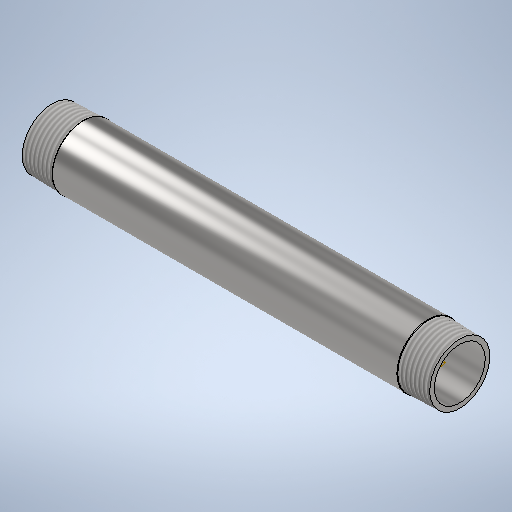
# Autodesk Inventor part: Threaded pipe_SGP._1ipt
Saved by Autodesk Inventor 2025.4 (Build 294407000, 407)
## iProperties
Created: 2026-06-08
Part Number: Threaded pipe_SGP._1ipt
Material: SS400
Document SubType Name: Modeling
Designer: huma2
Density: 7.98 g/cm^3
Appearance: 半つや出し
Manager: A_Shiramizu
Company: Eiko Engineering
length: 150.000 mm
Author: huma2
length: 200.000 mm
Comments: 免責事項 本3Dモデルは設計検討・参考用データです。寸法、形状、強度、材質、規格適合性、使用目的への適合性は保証しません。実際の設計・製作・使用にあたっては、利用者の責任でメーカー資料、規格、法令、現物確認、強度確認等を行ってください。 本データの使用・改変・流用・再配布により生じた損害、事故、不具合等について、作成者は一切責任を負いません。 Disclaimer This 3D model and related data are provided for reference and design study purposes only. The creator makes no warranty regarding dimensions, geometry, strength, material, standards compliance, or fitness for any particular purpose. Before actual design, fabrication, installation, purchase, or use, the user must verify all information, including actual products, manufacturer data, applicable standards, laws, and strength calculations. The creator shall not be liable for any damage, accident, defect, loss, or trouble arising from the use, modification, reuse, or redistribution of this data. Use of this data is entirely at the user's own risk.
Autodesk Inventor part; units mm, degrees
ref_plane "YZ Plane" through (0, 0, 0) normal (1, 0, 0) x (0, 1, 0)
ref_plane "XZ Plane" through (0, 0, 0) normal (0, 1, 0) x (-1, 0, 0)
ref_plane "XY Plane" through (0, 0, 0) normal (0, 0, 1) x (1, 0, 0)
sketch "スケッチ1" plane through (0, 0, 0) normal (0, 0, 1) x (1, 0, 0)
  line L0 (-110.39, 0) -> (110.39, 0)
  line L1 (-110.39, 0) -> (-110.39, 17)
  line L2 (-110.39, 17) -> (110.39, 17)
  line L3 (110.39, 0) -> (110.39, 17)
  line L4 (-110.39, 13.8) -> (110.39, 13.8)
  point P0 (0, 0)
  point P1 (0, 0)
  dimension "d0" = 34
  dimension "d1" = 3.2
  dimension "d2" = 220.78
  constraints: 10 end point, 2 point on line, 2 vertical, 1 coincident, 1 horizontal, 1 midpoint, 1 parallel
  measures "d0" diameter of L2 L0
  measures "d1" distance between parallel lines of L4 L2
  measures "d2" distance between parallel lines of L3 L1
revolve "回転1" add sketch "スケッチ1" angle 360 about axis through (-110.39, 0, 0) along (1, 0, 0) contours L1 L2 L3 L4
sketch "スケッチ2" plane through (0, 0, 0) normal (0, 0, 1) x (1, 0, 0)
  line L0 (-110.39, 17) -> (110.39, 17) projected
  line L1 (-110.39, -17) -> (-110.39, 17) projected
  line L2 (-110.39, 16.2998) -> (-93.6, 16.8245)
  line L3 (-93.6, 16.8245) -> (-93.296, 17)
  line L4 (-110.39, 0) -> (57.6085, 0)
  line L5 (-100, 16.6245) -> (-100, 0) construction
  point P0 (0, 0)
  dimension "d4" = 33.249
  dimension "d5" = 1.79
  dimension "d6" = 10.39
  dimension "d9" = 30
  dimension "d10" = 6.4
  constraints: 8 end point, 4 point on line, 1 horizontal, 1 midpoint, 1 perpendicular
  measures "d4" diameter of L5.start L4
  measures "d5" angle of L4 L2
  measures "d6" distance between parallel lines of L1 L5
  measures "d9" angle of L4 L3
  measures "d10" distance from line of L5 L2.end
revolve "回転2" cut sketch "スケッチ2" angle 360 about axis through (-110.39, 0, 0) along (1, 0, 0)
thread "ねじ1【手修正】" size "R 1" standard "JIS Taper" length 22.6
mirror "ミラー1" about plane through (0, 0, 0) normal (1, 0, 0) of "回転2"
thread "ねじ2【手修正】" size "R 1" standard "ISO Taper" length 23.2
ref_plane "作業平面1" through (-100, 0, 0) normal (-1, 0, 0) x (0, 0, 1)
ref_plane "作業平面2" through (100, 0, 0) normal (1, 0, 0) x (0, 0, -1)
equation "\"d0\" = DIA"
equation "\"d1\" = T1"
equation "\"d2\" = length + 2 * L1"
equation "\"d4\" = DIA_1"
equation "\"d6\" = L1"
equation "\"d10\" = L2"
equation "\"DIA\" = 34"
equation "\"T1\" = 3.2"
equation "\"DIA_1\" = 33.249"
equation "\"L1\" = 10.39"
equation "\"L2\" = 6.4"
equation "\"length\" = 200"
equation "\"d16\" = -L1"
equation "\"d17\" = -L1"
